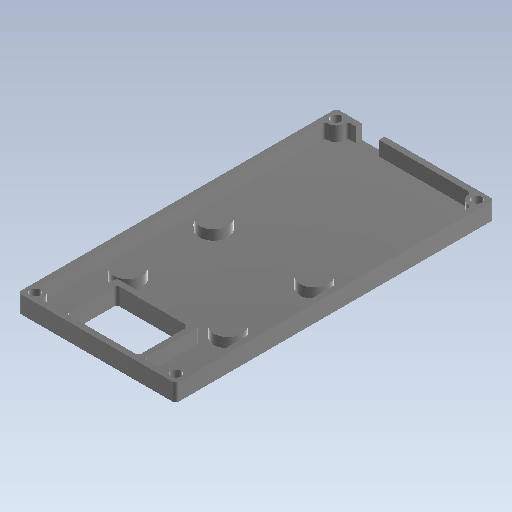
# Autodesk Inventor part: MainBoard_cover
Saved by Autodesk Inventor 2020 (Build 240168000, 168)
## iProperties
Created: 2021-05-13
Part Number: MainBoard_cover
Material: アセタール樹脂、黒
Document SubType Name: Modeling
Designer: Masato Kubotera
Density: 1.425 g/cm^3
Appearance: 滑らか - 黒
Mass: 13.7694 g
Surface Area: 157.492 cm^2
Volume: 9.66276 cm^3
Description: PLA
Author: Masato Kubotera
Title: Circuit_protection_01
Autodesk Inventor part; units mm, degrees
ref_plane "YZ Plane" through (0, 0, 0) normal (1, 0, 0) x (0, 1, 0)
ref_plane "XZ Plane" through (0, 0, 0) normal (0, 1, 0) x (-1, 0, 0)
ref_plane "XY Plane" through (0, 0, 0) normal (0, 0, 1) x (1, 0, 0)
derived "Cockpit_upper_bottom_frame.ipt"
sketch "スケッチ1" plane through (0, 0, 0) normal (0, 0, 1) x (1, 0, 0)
  line L0 (-32.25, 65) -> (32.25, 65) construction
  line L1 (32.25, 65) -> (32.25, 47.1) construction
  line L2 (-32.25, -65) -> (-32.25, -47.1) construction
  line L3 (-32.25, 65) -> (32.25, -65) construction
  line L4 (32.25, 65) -> (-32.25, -65) construction
  line L5 (-32.25, 45) -> (-37.25, 45) construction
  line L6 (-37.25, 15) -> (-32.25, 15) construction
  line L7 (-37.25, 15) -> (-37.25, 45) construction
  line L8 (-32.25, -15) -> (-37.25, -15) construction
  line L9 (-37.25, -15) -> (-37.25, -45) construction
  line L10 (-37.25, -45) -> (-32.25, -45) construction
  arc A0 (-32.25, 45) -> (-32.25, 47.1) centre (-32.25, 46.05) ccw construction
  arc A1 (-32.25, 12.9) -> (-32.25, 15) centre (-32.25, 13.95) ccw construction
  arc A2 (-32.25, -15) -> (-32.25, -12.9) centre (-32.25, -13.95) ccw construction
  arc A3 (-32.25, -47.1) -> (-32.25, -45) centre (-32.25, -46.05) ccw construction
  line L11 (-32.25, 47.1) -> (-32.25, 65) construction
  line L12 (-32.25, 12.9) -> (-32.25, 15) construction
  line L13 (-32.25, -12.9) -> (-32.25, 12.9) construction
  line L14 (-32.25, -47.1) -> (-32.25, -45) construction
  line L15 (0, 65) -> (0, -65) construction
  arc A4 (32.25, -45) -> (32.25, -47.1) centre (32.25, -46.05) ccw construction
  line L16 (37.25, -45) -> (32.25, -45) construction
  line L17 (37.25, -15) -> (37.25, -45) construction
  line L18 (32.25, -15) -> (37.25, -15) construction
  arc A5 (32.25, -12.9) -> (32.25, -15) centre (32.25, -13.95) ccw construction
  arc A6 (32.25, 15) -> (32.25, 12.9) centre (32.25, 13.95) ccw construction
  line L19 (37.25, 15) -> (37.25, 45) construction
  line L20 (37.25, 15) -> (32.25, 15) construction
  line L21 (32.25, 45) -> (37.25, 45) construction
  arc A7 (32.25, 47.1) -> (32.25, 45) centre (32.25, 46.05) ccw construction
  line L22 (32.25, 47.1) -> (32.25, 45) construction
  line L23 (32.25, 12.9) -> (32.25, -12.9) construction
  line L24 (32.25, -47.1) -> (32.25, -65) construction
  line L25 (32.25, -12.9) -> (32.25, -15) construction
  line L26 (-32.25, -15) -> (-32.25, -12.9) construction
  line L27 (-32.25, -45) -> (-32.25, -15) construction
  line L28 (32.25, -15) -> (32.25, -45) construction
  line L29 (32.25, -45) -> (32.25, -47.1) construction
  line L30 (-20, -11.25) -> (-15, -11.25) construction
  line L31 (-15, -11.25) -> (-15, -31.25) construction
  line L32 (-15, -31.25) -> (-20, -31.25) construction
  line L33 (-20, -31.25) -> (-20, -11.25) construction
  line L34 (-20, -11.25) -> (-15, -31.25) construction
  line L35 (-15, -11.25) -> (-20, -31.25) construction
  line L36 (-20, 2.5) -> (-15, 2.5) construction
  line L37 (-15, 2.5) -> (-15, -45) construction
  line L38 (-15, -45) -> (-20, -45) construction
  line L39 (-20, -45) -> (-20, 2.5) construction
  line L40 (-20, 2.5) -> (-15, -45) construction
  line L41 (-15, 2.5) -> (-20, -45) construction
  circle A8 centre (-17.5, -36.25) radius 1.55 construction
  line L42 (-20, -21.25) -> (-15, -21.25) construction
  line L43 (-17.5, 2.5) -> (-17.5, -45) construction
  circle A9 centre (-17.5, -6.25) radius 1.55 construction
  circle A10 centre (17.5, -6.25) radius 1.55 construction
  circle A11 centre (17.5, -36.25) radius 1.55 construction
  line L44 (32.25, -65) -> (16.75, -65) construction
  line L45 (-12.5, -62.5) -> (-12.5, -45) construction
  line L46 (-12.5, -45) -> (0, -45) construction
  line L47 (12.5, -45) -> (0, -45) construction
  line L48 (12.5, -62.5) -> (12.5, -45) construction
  line L49 (-16.75, -65) -> (-32.25, -65) construction
  line L50 (16.75, -65) -> (-16.75, -65) construction
  line L51 (-32.25, 45) -> (-32.25, 47.1) construction
  line L52 (-32.25, 15) -> (-32.25, 45) construction
  line L53 (32.25, 15) -> (32.25, 12.9) construction
  line L54 (32.25, 45) -> (32.25, 15) construction
  circle A12 centre (-24.5, 43.5) radius 1.25 construction
  line L55 (-32.25, 0) -> (32.25, 0) construction
  line L56 (-32.25, 46.5) -> (32.25, 46.5) construction
  circle A13 centre (-24.5, -61.5) radius 1.25 construction
  circle A14 centre (24.5, 43.5) radius 1.25 construction
  circle A15 centre (24.5, -61.5) radius 1.25 construction
  circle A16 centre (-17.5, -36.25) radius 3 construction
  line L57 (-27.5, 46.5) -> (27.5, 46.5)
  line L58 (27.5, -64.5) -> (-27.5, -64.5)
  line L59 (-27.5, -64.5) -> (-27.5, 46.5)
  circle A17 centre (-24.5, -61.5) radius 1.75
  arc A18 (-21.6716, -62.5) -> (-25.5, -58.6716) centre (-24.5, -61.5) ccw
  circle A19 centre (24.5, -61.5) radius 1.75
  arc A20 (25.5, -58.6716) -> (21.6716, -62.5) centre (24.5, -61.5) ccw
  circle A21 centre (-17.5, -6.25) radius 3
  circle A22 centre (-17.5, -6.25) radius 5
  circle A23 centre (-17.5, -36.25) radius 3
  circle A24 centre (17.5, -6.25) radius 3
  circle A25 centre (17.5, -6.25) radius 5
  circle A26 centre (17.5, -36.25) radius 3
  line L60 (-12.5, -62.5) -> (-12.5, -45)
  line L61 (-12.5, -45) -> (12.5, -45)
  line L62 (21.6716, -62.5) -> (14.5, -62.5)
  line L63 (-14.5, -62.5) -> (-21.6716, -62.5)
  line L64 (12.5, -62.5) -> (12.5, -45)
  line L65 (-14.5, -43) -> (-14.5, -62.5)
  line L66 (-14.5, -43) -> (14.5, -43)
  line L67 (14.5, -43) -> (14.5, -62.5)
  line L68 (-25.5, -58.6716) -> (-25.5, 40.6716)
  line L69 (27.5, -64.5) -> (27.5, 46.5)
  line L70 (25.5, -58.6716) -> (25.5, 40.6716)
  line L71 (-27.5, -9) -> (27.5, -9) construction
  circle A27 centre (-24.5, 43.5) radius 1.75
  arc A28 (-25.5, 40.6716) -> (-21.6716, 44.5) centre (-24.5, 43.5) ccw
  circle A29 centre (24.5, 43.5) radius 1.75
  arc A30 (21.6716, 44.5) -> (25.5, 40.6716) centre (24.5, 43.5) ccw
  line L72 (-21.6716, 44.5) -> (21.6716, 44.5)
  circle A31 centre (-17.5, -36.25) radius 5
  circle A32 centre (17.5, -36.25) radius 5
  line L73 (-12.5, -62.5) -> (12.5, -62.5)
  line L74 (-18.605, 46.5) -> (-18.605, 44.5)
  line L75 (-14.605, 46.5) -> (-14.605, 44.5) construction
  line L76 (-10.605, 46.5) -> (-10.605, 44.5)
  line L77 (-12.5, -62.5) -> (12.5, -62.5)
  line L78 (-24.25, 41.5) -> (24.25, 41.5)
  line L79 (24.25, 2.5) -> (-24.25, 2.5)
  line L80 (-24.25, 2.5) -> (-24.25, 41.5)
  line L81 (24.25, 2.5) -> (24.25, 41.5)
  line L82 (-20.05, -29.8151) -> (-18.5651, -31.3) construction
  line L83 (-19.3075, -30.5575) -> (-20.05, -31.3) construction
  arc A33 (-20.05, -29.8151) -> (-18.5651, -31.3) centre (-19.3075, -30.5575) ccw
  line L84 (-20.05, -11.2) -> (-18.5651, -11.2) construction
  line L85 (-14.95, -11.2) -> (-14.95, -12.6849) construction
  line L86 (-14.95, -31.3) -> (-16.4349, -31.3) construction
  line L87 (-20.05, -31.3) -> (-20.05, -29.8151) construction
  line L88 (-20.05, -11.2) -> (-14.95, -31.3) construction
  line L89 (-14.95, -11.2) -> (-20.05, -31.3) construction
  arc A34 (-16.4349, -31.3) -> (-14.95, -29.8151) centre (-15.6925, -30.5575) ccw
  arc A35 (-14.95, -12.6849) -> (-16.4349, -11.2) centre (-15.6925, -11.9425) ccw
  arc A36 (-18.5651, -11.2) -> (-20.05, -12.6849) centre (-19.3075, -11.9425) ccw
  line L90 (-20.05, -29.8151) -> (-20.05, -12.6849)
  line L91 (-18.5651, -31.3) -> (-20.05, -31.3) construction
  line L92 (-16.4349, -31.3) -> (-18.5651, -31.3)
  line L93 (-14.95, -29.8151) -> (-14.95, -31.3) construction
  line L94 (-20.05, -12.6849) -> (-20.05, -11.2) construction
  line L95 (-18.5651, -11.2) -> (-16.4349, -11.2)
  line L96 (-16.4349, -11.2) -> (-14.95, -11.2) construction
  line L97 (-14.95, -12.6849) -> (-14.95, -29.8151)
  arc A37 (14.95, -29.8151) -> (16.4349, -31.3) centre (15.6925, -30.5575) ccw
  line L98 (16.4349, -31.3) -> (18.5651, -31.3)
  arc A38 (18.5651, -31.3) -> (20.05, -29.8151) centre (19.3075, -30.5575) ccw
  line L99 (20.05, -29.8151) -> (20.05, -12.6849)
  line L100 (14.95, -12.6849) -> (14.95, -29.8151)
  arc A39 (20.05, -12.6849) -> (18.5651, -11.2) centre (19.3075, -11.9425) ccw
  line L101 (18.5651, -11.2) -> (16.4349, -11.2)
  arc A40 (16.4349, -11.2) -> (14.95, -12.6849) centre (15.6925, -11.9425) ccw
  line L102 (-32.25, -65) -> (-32.25, -70)
  line L103 (-32.25, -70) -> (32.25, -70)
  line L104 (32.25, -70) -> (32.25, -65)
  point P0 (0, 0)
  point P1 (0, 0)
  point P2 (0, 0)
  point P3 (-17.5, -21.25)
  point P4 (20.3453, -61)
  point P5 (25.5, 40.6716)
  point P6 (-12.5, -64.5)
  point P7 (-12.5, -46.25)
  point P8 (-14.5, -50.25)
  point P9 (14.5, -50.25)
  point P10 (12.5, -46.25)
  point P11 (12.5, -64.5)
  point P12 (-14.5, -51)
  point P13 (14.5, -51)
  point P14 (28, 15)
  point P15 (28, 45)
  point P16 (28, 45)
  point P17 (28, 15)
  point P18 (28, 15)
  point P19 (28, 45)
  point P20 (28, 45)
  point P21 (28, 15)
  point P22 (-22.5, -55.0139)
  point P23 (22.5, -55.0139)
  point P24 (21.2997, -58.25)
  point P25 (21.5717, -57.9019)
  point P26 (-21.2997, -58.25)
  point P27 (-21.5717, -57.9019)
  point P28 (-13.7003, -43)
  point P29 (13.7003, -43)
  dimension "d27" = 3.5
  dimension "d32" = 6
  dimension "d33" = 6
  dimension "d34" = 10
  dimension "d35" = 0
  dimension "d36" = 0
  dimension "d39" = 2
  dimension "d40" = 2
  dimension "d49" = 2
  dimension "d50" = 2
  dimension "d55" = 14.605
  dimension "d56" = 8
  dimension "d57" = 3
  dimension "d58" = 3
  measures "d27" diameter of A17
  measures "d32" diameter of A18
  measures "d33" diameter of A21
  measures "d34" diameter of A22
  measures "d35" distance between parallel lines of L45 L60
  measures "d36" distance between parallel lines of L61 L46
  measures "d39" distance between parallel lines of L65 L60
  measures "d40" distance between parallel lines of L61 L66
  measures "d49" distance between parallel lines of L59 L68
  measures "d50" distance between parallel lines of L58 L63
  measures "d55" distance between parallel lines of L15 L75
  measures "d56" distance between parallel lines of L74 L76
  measures "d57" distance from line of L59 A28.centre
  measures "d58" distance from line of L58 A13.centre
extrude "押し出し1" add sketch "スケッチ1" along normal blind 6 contours L57 L74 L72 A28 L78 L80 L68 A18 L63 L65 L66 L67 L62 A20 L70 A30 L81 L76 L69 L58 L59 | A28 L80 L78 | L78 L81 A30
extrude "押し出し2" add sketch "スケッチ1" along normal blind 1 contours L57 L76 L72 L74 | L72 A30 L78 A28 | L78 A30 L81 L79 L80 A28 | L80 L79 L81 A30 L70 A20 L62 L67 L66 L65 L63 A18 L68 A28 | A36 A22 | A22 A36 L95 A35 L97 A34 A31 L92 A33 L90 | A22 A35 | A22 L95 A36 | A35 L95 A22 | L95 A22 | A33 A31 L92 A34 | A31 A33 | A34 A31 | A33 L92 A31 | A31 L92 A34 | A31 L92 | A23 | A40 A25 | A25 A40 L101 A39 L99 A38 A32 L98 A37 L100 | A25 A39 | A25 L101 A40 | A39 L101 A25 | L101 A25 | A37 A32 L98 A38 | A32 A37 | A38 A32 | A37 L98 A32 | A32 L98 A38 | A32 L98 | A26
extrude "押し出し3" add sketch "スケッチ1" along normal blind 4.4 contours A21 | A22 A35 L95 A36 | A36 A22 | A22 A35 | L95 A22 | A33 A31 L92 A34 | A31 A33 | A34 A31 | A31 L92 | A23 | A24 | A25 A39 L101 A40 | A40 A25 | A25 A39 | L101 A25 | A37 A32 L98 A38 | A32 A37 | A38 A32 | A32 L98 | A26
extrude "押し出し4" cut sketch "スケッチ1" along normal blind 3.5 contours A21 | A23 | A24 | A26
fillet "フィレット1" radius 1 20 edges at (21.6716, -62.5, 3.5) (14.5, -43, 3.5) (-21.6716, -62.5, 3.5) (-25.5, -58.6716, 3.5) (-14.5, -43, 3.5) (14.5, -62.5, 3.5) (-14.5, -62.5, 3.5) (-27.5, -64.5, 3) (-12.5, -45, 3) (12.5, -45, 3) (12.5, -62.5, 3) (27.5, -64.5, 3) (25.5, -58.6716, 3.5) (-27.5, 46.5, 3) (-25.5, 40.6716, 3.5) (-21.6716, 44.5, 3.5) (25.5, 40.6716, 3.5) (21.6716, 44.5, 3.5) (27.5, 46.5, 3) (-12.5, -62.5, 3)
equation "\"d39\" = d50"
equation "\"d40\" = d50"
equation "\"d50\" = d49"
equation "\"d19\" = d18"
equation "\"d18\" = 2"
